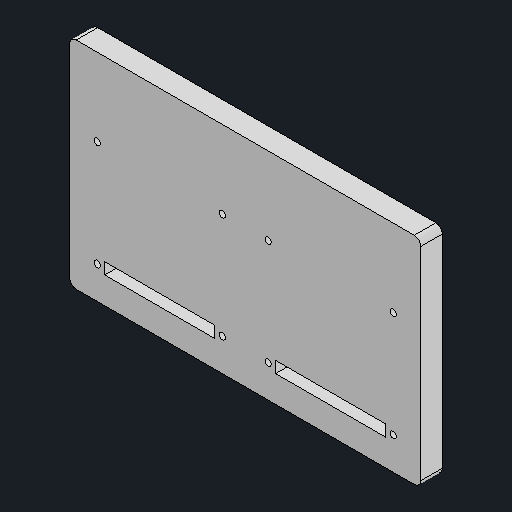
# Autodesk Inventor part: RasPi-Hat-outline
Saved by Autodesk Inventor 2026 (Build 300175050, 175E)
## iProperties
Created: 2025-08-29
Part Number: RasPi-Hat-outline
Material: Generic
Document SubType Name: Modeling
Designer: queezz
Density: 1 g/cm^3
Appearance: Default
Author: queezz
Autodesk Inventor part; units mm, degrees
ref_plane "YZ Plane" through (0, 0, 0) normal (1, 0, 0) x (0, 1, 0)
ref_plane "XZ Plane" through (0, 0, 0) normal (0, 1, 0) x (-1, 0, 0)
ref_plane "XY Plane" through (0, 0, 0) normal (0, 0, 1) x (1, 0, 0)
sketch "Sketch1" plane through (0, 0, 0) normal (0, 0, 1) x (1, 0, 0)
  line L0 (-81.3375, 50) -> (81.3375, 50)
  line L1 (81.3375, 50) -> (81.3375, -50)
  line L2 (81.3375, -50) -> (-81.3375, -50)
  line L3 (-81.3375, -50) -> (-81.3375, 50)
  point P0 (0, 0)
  point P1 (0, 50)
  point P2 (81.3375, 0)
  dimension "d0" = 100
  dimension "d1" = 162.675
  constraints: 8 end point, 2 midpoint, 2 parallel, 1 horizontal, 1 horizontal alignment, 1 perpendicular, 1 vertical alignment
  measures "d0" distance of L0.end L1.end
  measures "d1" distance of L0.start L0.end
extrude "Extrusion1" add sketch "Sketch1" along normal blind 10
sketch "Sketch2" plane through (0, 0, 10) normal (0, 0, 1) x (1, 0, 0)
  line L0 (10.6002, 14) -> (68.6002, 14) construction
  line L1 (68.6002, 14) -> (68.6002, -35) construction
  line L2 (68.6002, -35) -> (10.6002, -35) construction
  line L3 (10.6002, -35) -> (10.6002, 14) construction
  line L4 (-81.3375, -50) -> (81.3375, -50) projected
  point P0 (0, 0)
  dimension "d4" = 58
  dimension "d5" = 49
  dimension "d18" = 15
  constraints: 8 end point, 4 coincident, 2 parallel, 1 horizontal, 1 perpendicular
  measures "d4" distance of L0.start L0.end
  measures "d5" distance of L0.end L1.end
  measures "d18" distance between parallel lines of L4 L2
hole "Hole1" at (10.6002, 14, 10) at (68.6002, 14, 10) at (68.6002, -35, 10) at (10.6002, -35, 10) direction (0, 0, -1) diameter 3 end through all
sketch "Sketch3" plane through (0, 0, 10) normal (0, 0, 1) x (1, 0, 0)
  line L0 (14.1002, -32.35) -> (65.1002, -32.35)
  line L1 (65.1002, -32.35) -> (65.1002, -37.65)
  line L2 (65.1002, -37.65) -> (14.1002, -37.65)
  line L3 (14.1002, -37.65) -> (14.1002, -32.35)
  circle A0 centre (68.6002, -35) radius 1.5 projected
  circle A1 centre (10.6002, -35) radius 1.5 projected
  line L4 (10.6002, -35) -> (68.6002, -35) construction
  point P0 (0, 0)
  point P1 (65.1002, -35)
  point P2 (39.6002, -35)
  point P3 (39.6002, -32.35)
  dimension "d14" = 5.3
  dimension "d15" = 51
  constraints: 10 end point, 3 midpoint, 2 horizontal, 2 parallel, 1 horizontal alignment, 1 perpendicular, 1 vertical alignment
  measures "d14" distance of L0.end L1.end
  measures "d15" distance of L0.start L0.end
extrude "Extrusion2" cut sketch "Sketch3" against normal through all contours L0 L1 L2 L3
mirror "Mirror1" about plane through (0, 0, 0) normal (1, 0, 0) of "Hole1", "Extrusion2"
fillet "Fillet1" radius 3 4 edges at (81.3375, 50, 5) (-81.3375, 50, 5) (-81.3375, -50, 5) (81.3375, -50, 5)
equation "\"d1\" = 2.5 * width"
equation "\"hight\" = 56.21"
equation "\"width\" = 65.07"
body "Solid1"
